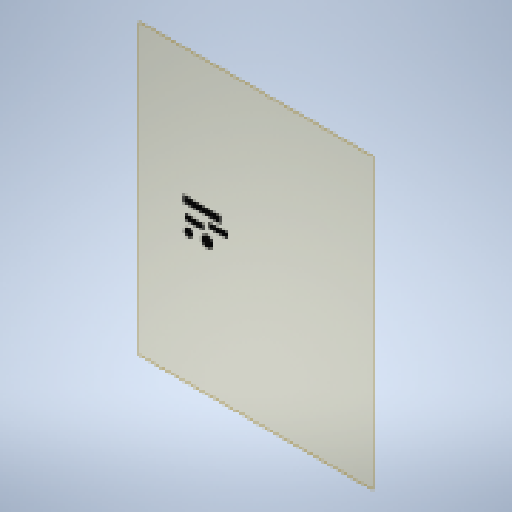
# Autodesk Inventor part: on-air-control-layout-2
Saved by Autodesk Inventor 2023 (Build 270158030, 158C)
## iProperties
Created: 2024-04-02
Part Number: on-air-control-layout-2
Material: Generic
Document SubType Name: Modeling
Designer: Imogen Heard
Density: 1 g/cm^3
Appearance: Default
Author: Imogen Heard
Autodesk Inventor part; units mm, degrees
ref_plane "YZ Plane" through (0, 0, 0) normal (1, 0, 0) x (0, 1, 0)
ref_plane "XZ Plane" through (0, 0, 0) normal (0, 1, 0) x (-1, 0, 0)
ref_plane "XY Plane" through (0, 0, 0) normal (0, 0, 1) x (1, 0, 0)
ref_plane "Work Plane1" through (0, 0, 0) normal (0, 0, 1) x (1, 0, 0)
sketch "Sketch1" plane through (0, 0, 0) normal (0, 0, 1) x (1, 0, 0)
  line L0 (-135.1554, 30.9947) -> (-65.1554, 30.9947)
  line L1 (-65.1554, 30.9947) -> (-65.1554, 18.9947)
  line L2 (-65.1554, 18.9947) -> (-135.1554, 18.9947)
  line L3 (-135.1554, 18.9947) -> (-135.1554, 30.9947)
  circle A0 centre (-125.1554, -25.0053) radius 8
  circle A1 centre (-125.1554, -25.0053) radius 10 construction
  circle A2 centre (-90.1554, -22.5053) radius 11
  circle A3 centre (-90.1554, -22.5053) radius 14.5 construction
  line L4 (-132.1554, 2.4947) -> (-97.1554, 2.4947)
  line L5 (-97.1554, 2.4947) -> (-97.1554, -7.5053)
  line L6 (-97.1554, -7.5053) -> (-132.1554, -7.5053)
  line L7 (-132.1554, -7.5053) -> (-132.1554, 2.4947)
  line L8 (-88.1554, 10.9947) -> (-53.1554, 10.9947)
  line L9 (-53.1554, 10.9947) -> (-53.1554, 0.9947)
  line L10 (-53.1554, 0.9947) -> (-88.1554, 0.9947)
  line L11 (-88.1554, 0.9947) -> (-88.1554, 10.9947)
  point P0 (0, 0)
  dimension "d0" = 70
  dimension "d1" = 12
  dimension "d2" = 16
  dimension "d3" = 20
  dimension "d4" = 22
  dimension "d5" = 29
  dimension "d6" = 10
  dimension "d7" = 35
  dimension "d8" = 10
  dimension "d9" = 35
  dimension "d10" = 3
  dimension "d11" = 8.5
  dimension "d12" = 25
  dimension "d13" = 2.5
  dimension "d14" = 35
  dimension "d15" = 9
  dimension "d16" = 20
  dimension "d17" = 15
  constraints: 24 end point, 6 parallel, 4 centre point, 3 horizontal, 3 perpendicular, 1 coincident
  measures "d0" distance between parallel lines of L1 L3
  measures "d1" distance between parallel lines of L2 L0
  measures "d2" diameter of A0
  measures "d3" diameter of A1
  measures "d4" diameter of A2
  measures "d5" diameter of A3
  measures "d6" distance between parallel lines of L6 L4
  measures "d7" distance between parallel lines of L7 L5
  measures "d8" distance between parallel lines of L10 L8
  measures "d9" distance between parallel lines of L11 L9
  measures "d10" distance from line of L0.start L7
  measures "d11" distance between parallel lines of L4 L8
  measures "d12" distance from line of L1 A2.centre
  measures "d13" vertical distance of A0.centre A2.centre
  measures "d14" horizontal distance of A2.centre A0.centre
  measures "d15" distance between parallel lines of L11 L5
  measures "d16" distance between parallel lines of L8 L0
  measures "d17" distance from line of A2.centre L6
extrude "Extrusion1" add sketch "Sketch1" along normal blind 1
sketch "Sketch2" plane through (0, 0, 1) normal (0, 0, 1) x (1, 0, 0)
  line L0 (-133.486, 28.5794) -> (-66.3333, 28.5794) construction
  line L1 (-66.3333, 28.5794) -> (-66.3333, 21.4782) construction
  line L2 (-66.3333, 21.4782) -> (-133.486, 21.4782) construction
  line L3 (-133.486, 21.4782) -> (-133.486, 28.5794) construction
  point P0 (0, 0)
  constraints: 1 horizontal alignment, 2 other
decal "Decal1"
body "Solid1"
